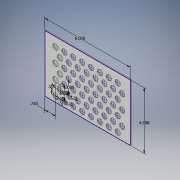
# Autodesk Inventor part: FlaperWithHoles
Saved by Autodesk Inventor 2017 (Build 210142000, 142)
## iProperties
Created: 2017-11-11
Part Number: FlaperWithHoles
Material: Generic
Document SubType Name: Modeling
Designer: User
Density: 1 g/cm^3
Appearance: Default
Author: User
Autodesk Inventor part; units mm, degrees
ref_plane "YZ Plane" through (0, 0, 0) normal (1, 0, 0) x (0, 1, 0)
ref_plane "XZ Plane" through (0, 0, 0) normal (0, 1, 0) x (-1, 0, 0)
ref_plane "XY Plane" through (0, 0, 0) normal (0, 0, 1) x (1, 0, 0)
sketch "Sketch1" plane through (0, 0, 0) normal (0, 0, 1) x (1, 0, 0)
  line L0 (0, 0) -> (152.4, 0)
  line L1 (152.4, 0) -> (152.4, 101.6)
  line L2 (152.4, 101.6) -> (0, 101.6)
  line L3 (0, 101.6) -> (0, 0)
  point P0 (19.05, 9.525)
  point P1 (34.925, 9.525)
  point P2 (50.8, 9.525)
  point P3 (66.675, 9.525)
  point P4 (82.55, 9.525)
  point P5 (98.425, 9.525)
  point P6 (114.3, 9.525)
  point P7 (130.175, 9.525)
  point P8 (26.9875, 22.225)
  point P9 (42.8625, 22.225)
  point P10 (58.7375, 22.225)
  point P11 (74.6125, 22.225)
  point P12 (90.4875, 22.225)
  point P13 (106.3625, 22.225)
  point P14 (122.2375, 22.225)
  point P15 (138.1125, 22.225)
  point P16 (50.8, 9.525)
  point P17 (66.675, 9.525)
  point P18 (82.55, 9.525)
  point P19 (98.425, 9.525)
  point P20 (114.3, 9.525)
  point P21 (130.175, 9.525)
  point P22 (34.925, 34.925)
  point P23 (50.8, 34.925)
  point P24 (66.675, 34.925)
  point P25 (82.55, 34.925)
  point P26 (98.425, 34.925)
  point P27 (114.3, 34.925)
  point P28 (130.175, 34.925)
  point P29 (34.925, 60.325)
  point P30 (50.8, 60.325)
  point P31 (66.675, 60.325)
  point P32 (82.55, 60.325)
  point P33 (98.425, 60.325)
  point P34 (114.3, 60.325)
  point P35 (130.175, 60.325)
  point P36 (34.925, 85.725)
  point P37 (50.8, 85.725)
  point P38 (66.675, 85.725)
  point P39 (82.55, 85.725)
  point P40 (98.425, 85.725)
  point P41 (114.3, 85.725)
  point P42 (130.175, 85.725)
  point P43 (58.7375, 22.225)
  point P44 (74.6125, 22.225)
  point P45 (90.4875, 22.225)
  point P46 (106.3625, 22.225)
  point P47 (122.2375, 22.225)
  point P48 (138.1125, 22.225)
  point P49 (42.8625, 47.625)
  point P50 (58.7375, 47.625)
  point P51 (74.6125, 47.625)
  point P52 (90.4875, 47.625)
  point P53 (106.3625, 47.625)
  point P54 (122.2375, 47.625)
  point P55 (138.1125, 47.625)
  point P56 (42.8625, 73.025)
  point P57 (58.7375, 73.025)
  point P58 (74.6125, 73.025)
  point P59 (90.4875, 73.025)
  point P60 (106.3625, 73.025)
  point P61 (122.2375, 73.025)
  point P62 (138.1125, 73.025)
  point P63 (19.05, 34.925)
  point P64 (19.05, 60.325)
  point P65 (19.05, 85.725)
  point P66 (26.9875, 47.625)
  point P67 (26.9875, 73.025)
  dimension "d0" = 152.4
  dimension "d1" = 101.6
  dimension "d2" = 9.525
  dimension "d3" = 19.05
  dimension "d6" = 15.875
  dimension "d11" = 12.7
  dimension "d12" = 7.9375
  dimension "d15" = 15.875
  dimension "d22" = 15.875
  dimension "d25" = 25.4
  dimension "d30" = 15.875
  dimension "d33" = 25.4
  constraints: 8 end point, 5 horizontal, 2 parallel, 2 vertical, 1 perpendicular, 61 other
  measures "d0" distance of L1.end L2.end
  measures "d1" distance of L0.end L1.end
  measures "d2" distance from line of L0 point (19.05, 9.525)
  measures "d3" distance from line of point (19.05, 9.525) L3
  measures "d6" distance of point (19.05, 9.525) point (34.925, 9.525)
  measures "d11" vertical distance of point (26.988, 22.225) point (19.05, 9.525)
  measures "d12" horizontal distance of point (26.988, 22.225) point (19.05, 9.525)
  measures "d15" distance of point (26.988, 22.225) point (42.862, 22.225)
  measures "d22" distance of point (34.925, 9.525) point (50.8, 9.525)
  measures "d25" distance of point (34.925, 9.525) point (34.925, 34.925)
  measures "d30" distance of point (42.862, 22.225) point (58.737, 22.225)
  measures "d33" distance of point (42.862, 22.225) point (42.862, 47.625)
extrude "Extrusion1" add sketch "Sketch1" against normal blind 1.524
hole "Hole1" at (19.05, 9.525, 0) at (34.925, 9.525, 0) at (50.8, 9.525, 0) at (66.675, 9.525, 0) at (82.55, 9.525, 0) at (98.425, 9.525, 0) at (114.3, 9.525, 0) at (130.175, 9.525, 0) at (26.9875, 22.225, 0) at (42.8625, 22.225, 0) at (58.7375, 22.225, 0) at (74.6125, 22.225, 0) at (90.4875, 22.225, 0) at (106.3625, 22.225, 0) at (122.2375, 22.225, 0) at (138.1125, 22.225, 0) at (34.925, 34.925, 0) at (50.8, 34.925, 0) at (66.675, 34.925, 0) at (82.55, 34.925, 0) at (98.425, 34.925, 0) at (114.3, 34.925, 0) at (130.175, 34.925, 0) at (34.925, 60.325, 0) at (50.8, 60.325, 0) at (66.675, 60.325, 0) at (82.55, 60.325, 0) at (98.425, 60.325, 0) at (114.3, 60.325, 0) at (130.175, 60.325, 0) at (34.925, 85.725, 0) at (50.8, 85.725, 0) at (66.675, 85.725, 0) at (82.55, 85.725, 0) at (98.425, 85.725, 0) at (114.3, 85.725, 0) at (130.175, 85.725, 0) at (42.8625, 47.625, 0) at (58.7375, 47.625, 0) at (74.6125, 47.625, 0) at (90.4875, 47.625, 0) at (106.3625, 47.625, 0) at (122.2375, 47.625, 0) at (138.1125, 47.625, 0) at (42.8625, 73.025, 0) at (58.7375, 73.025, 0) at (74.6125, 73.025, 0) at (90.4875, 73.025, 0) at (106.3625, 73.025, 0) at (122.2375, 73.025, 0) direction (0, 0, -1) diameter 9.525 end through all and at (138.1125, 73.025, 0) (19.05, 34.925, 0) (19.05, 60.325, 0) (19.05, 85.725, 0) (26.9875, 47.625, 0) (26.9875, 73.025, 0)
equation "\"d12\" = 0.5 * d6"
body "Solid1"
